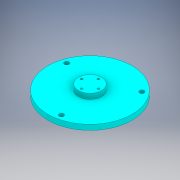
# Autodesk Inventor part: rotate_plate_4
Saved by Autodesk Inventor 2018 (Build 220112000, 112)
## iProperties
Created: 2019-01-16
Part Number: rotate_plate_4
Material: 一般
Document SubType Name: Modeling
Designer: lowyu
Density: 1 g/cm^3
Appearance: 既定
Author: lowyu
Autodesk Inventor part; units mm, degrees
ref_plane "YZ Plane" through (0, 0, 0) normal (1, 0, 0) x (0, 1, 0)
ref_plane "XZ Plane" through (0, 0, 0) normal (0, 1, 0) x (-1, 0, 0)
ref_plane "XY Plane" through (0, 0, 0) normal (0, 0, 1) x (1, 0, 0)
sketch "スケッチ1" plane through (0, 0, 0) normal (0, 0, 1) x (1, 0, 0)
  circle A0 centre (0, 0) radius 40
  circle A1 centre (26.1561, 23.2563) radius 2.1
  circle A2 centre (-33.2186, 11.0237) radius 2.1
  circle A3 centre (7.0625, -34.28) radius 2.1
  dimension "d0" = 80
  dimension "d3" = 4.2
  dimension "d4" = 35
  dimension "d7" = 360
  constraints: 4 centre point, 1 coincident, 7 other
  measures "d0" diameter of A0
  measures "d3" diameter of A1
  measures "d4" distance of A1.centre A0.centre
extrude "押し出し1" add sketch "スケッチ1" along normal blind 5 contours A0 | A1 | A2 | A3
sketch "スケッチ2" plane through (0, 0, 5) normal (0, 0, 1) x (1, 0, 0)
  circle A0 centre (0, 0) radius 40
  circle A1 centre (26.1561, 23.2563) radius 2.1
  circle A2 centre (-33.2186, 11.0237) radius 2.1
  circle A3 centre (7.0625, -34.28) radius 2.1
  dimension "d11" = 80
  dimension "d12" = 4.2
  dimension "d13" = 35
  dimension "d14" = 360
  constraints: 4 centre point, 1 coincident, 7 other
  measures "d11" diameter of A0
  measures "d12" diameter of A1
  measures "d13" distance of A1.centre A0.centre
extrude "押し出し2" cut sketch "スケッチ2" against normal blind 5 contours A1 | A2 | A3
sketch "スケッチ3" plane through (0, 0, 5) normal (0, 0, 1) x (1, 0, 0)
  circle A0 centre (0, 0) radius 11
  dimension "d17" = 22
  constraints: 1 centre point, 1 coincident
  measures "d17" diameter of A0
extrude "押し出し3" add sketch "スケッチ3" along normal blind 5
sketch "スケッチ4" plane through (0, 0, 10) normal (0, 0, 1) x (1, 0, 0)
  circle A0 centre (0, 8) radius 1
  line L0 (0, -56) -> (0, 56) projected
  circle A1 centre (-8, 0) radius 1
  circle A2 centre (0, -8) radius 1
  circle A3 centre (8, 0) radius 1
  point P0 (0, 0)
  dimension "d20" = 2
  dimension "d21" = 8
  dimension "d24" = 360
  constraints: 4 centre point, 1 point on line, 9 other
  measures "d20" diameter of A0
  measures "d21" distance of point (0, 0) A0.centre
extrude "押し出し4" cut sketch "スケッチ4" against normal blind 10
sketch "スケッチ5" plane through (0, 0, 0) normal (0, 0, -1) x (-1, 0, 0)
  circle A0 centre (-8, 0) radius 1 projected
  circle A1 centre (-8, 0) radius 1.9
  circle A2 centre (0, -8) radius 1.9
  circle A3 centre (8, 0) radius 1.9
  circle A4 centre (0, 8) radius 1.9
  point P0 (0, 0)
  dimension "d28" = 3.8
  dimension "d31" = 360
  constraints: 4 centre point, 1 coincident, 9 other
  measures "d28" diameter of A1
extrude "押し出し5" cut sketch "スケッチ5" against normal blind 1.8
